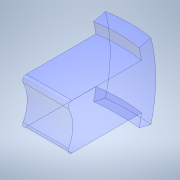
# Autodesk Inventor part: shank_2
Saved by Autodesk Inventor 2020.2 (Build 242310000, 310)
## iProperties
Created: 2021-01-30
Part Number: shank_2
Material: Generic
Document SubType Name: Modeling
Designer: DELL
Density: 1 g/cm^3
Appearance: Clear - Blue
Author: DELL
Autodesk Inventor part; units mm, degrees
ref_plane "XZ Plane" through (0, 0, 0) normal (0, 1, 0) x (-1, 0, 0)
ref_plane "XY Plane" through (0, 0, 0) normal (0, 0, 1) x (1, 0, 0)
ref_plane "UCS1: YZ Plane" through (0, 0, 0) normal (1, 0, 0) x (0, 1, 0)
sketch "Sketch17" plane through (0, 0, 0) normal (1, 0, 0) x (0, 1, 0)
  line L0 (-151.0923, 0) -> (102.6542, 0) construction
  line L1 (0, -203.2967) -> (0, 99.7801) projected
  circle A0 centre (0, 0) radius 40
  circle A1 centre (0, 0) radius 48.5
  arc A2 (-55.612, -135.6294) -> (55.612, -135.6294) centre (0, 56.4834) ccw
  arc A3 (-60, -150.7878) -> (60, -150.7878) centre (0, 40) ccw
  line L2 (55.612, -135.6294) -> (60, -150.7878)
  line L3 (-60, -150.7878) -> (-55.612, -135.6294)
  line L4 (-30, -38.1084) -> (-30, -143.5166)
  line L5 (-30, -143.5166) -> (30, -143.5166)
  line L6 (30, -143.5166) -> (30, -38.1084)
  line L7 (-46.1537, -138.1184) -> (-50, -153.6492)
  line L8 (46.1537, -138.1184) -> (50, -153.6492)
  line L9 (-50, -153.6492) -> (-28.9607, -159.0815) construction
  line L10 (-46.1537, -138.1184) -> (-25.0109, -143.1328) construction
  line L11 (-48.0768, -145.8838) -> (-13.8184, -154.3682) construction
  arc A4 (26.4209, -127.5166) -> (26, -143.5166) centre (66.4047, -136.574) ccw
  arc A5 (26.4209, -127.5166) -> (30, -95.5166) centre (-114.8428, -95.5166) ccw
  point P0 (0, -160)
  point P1 (0, -143.5166)
  point P2 (0, -160)
  point P3 (0, -48.5)
  point P4 (0, -143.5166)
  dimension "d173" = 97
  dimension "d174" = 80
  dimension "d224" = 60
  dimension "d229" = 160
  dimension "d230" = 200
  dimension "d231" = 15.7808
  dimension "d232" = 100
  dimension "d233" = 10
  dimension "d235" = 200
  dimension "d241" = 16
  dimension "d242" = 16.1537
  dimension "d243" = 16
  dimension "d244" = 32
  dimension "d245" = 26
  constraints: 20 end point, 16 point on circle, 6 centre point, 5 tangent, 4 point on line, 3 perpendicular, 2 coincident, 1 equal length, 1 line through centre, 1 midpoint, 1 vertical, 5 other
  measures "d173" diameter of A1
  measures "d174" diameter of A0
  measures "d224" distance of L4.end L5.end
  measures "d229" distance from line of point (0, -160) L0
  measures "d230" radius of A3
  measures "d231" distance of L2.start L2.end
  measures "d232" diameter of L7.end L1
  measures "d233" horizontal distance of L3.start L7.end
  measures "d235" radius of A2
  measures "d241" distance of L8.start L8.end
  measures "d242" distance from line of L6 L8.start
  measures "d243" vertical distance of A4.end A4.start
  measures "d244" vertical distance of A4.start A5.end
  measures "d245" distance from line of A4.end L1
sketch "Sketch16" plane through (0, 0, 0) normal (1, 0, 0) x (0, 1, 0)
  circle A0 centre (0, 0) radius 40
  circle A1 centre (0, 0) radius 48.5
  line L0 (0, -201.7) -> (0, 90.2) construction
  line L1 (0, -160) -> (0, -48.5)
  line L2 (30, -38.1084) -> (30, -103.6436)
  line L3 (30, -103.6436) -> (25, -132)
  line L4 (25, -132) -> (50, -132)
  line L5 (50, -132) -> (50, -160)
  line L6 (50, -160) -> (0, -160)
  dimension "d156" = 97
  dimension "d157" = 80
  dimension "d202" = 28
  dimension "d203" = 60
  dimension "d204" = 50
  dimension "d206" = 160
  dimension "d209" = 50
  dimension "d210" = 80
  dimension "d211" = 28.7938
  constraints: 12 end point, 2 centre point, 2 coincident, 2 horizontal, 2 point on circle, 2 point on line, 2 vertical
  measures "d156" diameter of A1
  measures "d157" diameter of A0
  measures "d202" distance of L4.end L5.end
  measures "d203" diameter of L2 L0
  measures "d204" distance of L5.end L1.start
  measures "d206" distance from line of point (0, 0) L6
  measures "d209" diameter of L3.end L0
  measures "d210" angle of L4 L3
  measures "d211" distance of L2.end L3.end
extrude "Extrusion14" [suppressed]
fillet "Fillet10" [suppressed]
mirror "Mirror1" [suppressed]
thicken "Thicken1" [suppressed]
sketch "Sketch19" plane through (0, 0, 0) normal (0, 1, 0) x (-1, 0, 0)
  arc A0 (-110.8458, -111.0605) -> (110.8458, -111.0605) centre (0, -10) ccw
  line L0 (155.1841, 0) -> (-155.1841, 0) projected
  line L1 (0, -264.129) -> (0, 44.0215) projected
  line L2 (110.8458, -111.0605) -> (110.8458, -220.1075)
  line L3 (110.8458, -220.1075) -> (-110.8458, -220.1075)
  line L4 (-110.8458, -220.1075) -> (-110.8458, -111.0605)
  point P0 (0, 0)
  point P1 (0, -160)
  point P2 (0, -160)
  point P3 (0, -220.1075)
  dimension "d217" = 150
  dimension "d218" = 0
  constraints: 6 end point, 3 point on circle, 2 point on line, 2 vertical, 1 centre point, 1 horizontal, 1 symmetric about line
  measures "d217" radius of A0
  measures "d218" distance of point (0, -160) point (0, -160)
revolve "Revolution1" [suppressed]
fillet "Fillet15" [suppressed]
revolve "Revolution2" add sketch "Sketch17" angle 360 about axis through (0, 0, -10) along (0, 0, 1) separate body contours L1 L5 L6 A2 L8 A3 | A2 A4 L5 | L8 A2 L2 A3 | A2 L6 L5 A4
ref_plane "Work Plane7" through (0, -46.1537, -138.1184) normal (0, -0.9706749, 0.240396) x (0, -0.240396, -0.9706749)
split "Split2" plane through (0, -46.1537, -138.1184) removes the side toward (0, -0.9706749, 0.240396)
ref_plane "Work Plane8" through (0, 46.1537, -138.1184) normal (0, -0.9706749, -0.240396) x (0, 0.240396, -0.9706749)
split "Split3" plane through (0, 46.1537, -138.1184) removes the side toward (0, 0.9706749, 0.240396)
ref_plane "Work Plane9" through (-30, 0, 0) normal (1, 0, 0) x (0, 1, 0)
split "Split4" plane through (-30, 0, 0) removes the side toward (-1, 0, 0)
ref_plane "Work Plane10" through (30, 0, 0) normal (1, 0, 0) x (0, 1, 0)
split "Split5" plane through (30, 0, 0) removes the side toward (1, 0, 0)
extrude "Extrusion17" add sketch "Sketch17" along normal mid plane 60 contours L1 A1 L6 A5 A4 A2 | A2 A4 L5 | A4 A5 L6 A2 | A2 L6 L5 A4
fillet "Fillet16" radius 5 1 edges at (0, 30, -38.1084)
mirror "Mirror4" about plane through (0, 0, 0) normal (0, 1, 0) of "Extrusion17", "Fillet16"
body "Solid1"
body "Solid6"
body "Solid8"
